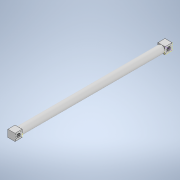
# Autodesk Inventor part: wał
Saved by Autodesk Inventor 2022 (Build 260153000, 153)
## iProperties
Created: 2023-04-25
Part Number: wał
Material: Ogólny
Document SubType Name: Modeling
Designer: nosal
Density: 1 g/cm^3
Appearance: Domyślna
Author: nosal
Autodesk Inventor part; units mm, degrees
ref_plane "YZ Plane" through (0, 0, 0) normal (1, 0, 0) x (0, 1, 0)
ref_plane "XZ Plane" through (0, 0, 0) normal (0, 1, 0) x (-1, 0, 0)
ref_plane "XY Plane" through (0, 0, 0) normal (0, 0, 1) x (1, 0, 0)
sketch "Szkic1" plane through (0, 0, 0) normal (0, 0, 1) x (1, 0, 0)
  circle A0 centre (0, 0) radius 4
  dimension "d0" = 8
  constraints: 1 centre point, 1 coincident
  measures "d0" diameter of A0
extrude "Wyciągnięcie proste1" add sketch "Szkic1" along normal blind 160
sketch "Szkic2" plane through (0, 0, 160) normal (0, 0, 1) x (1, 0, 0)
  line L0 (4, -4) -> (-4, -4)
  line L1 (-4, -4) -> (-4, 4)
  line L2 (-4, 4) -> (4, 4)
  line L3 (4, 4) -> (4, -4)
  line L4 (4, -4) -> (-4, 4) construction
  line L5 (-4, -4) -> (4, 4) construction
  point P0 (0, 0)
  dimension "d3" = 8
  dimension "d4" = 8
  constraints: 12 end point, 2 midpoint, 2 parallel, 1 horizontal, 1 perpendicular
  measures "d3" distance of L1.end L2.end
  measures "d4" distance of L0.end L1.end
extrude "Wyciągnięcie proste2" add sketch "Szkic2" along normal blind 8
sketch "Szkic3" plane through (0, 0, 0) normal (0, 0, -1) x (-1, 0, 0)
  line L0 (4, -4) -> (-4, -4) projected
  line L1 (4, 4) -> (-4, 4)
  line L2 (-4, 4) -> (-4, -4)
  line L3 (-4, -4) -> (4, -4)
  line L4 (4, -4) -> (4, 4)
  line L5 (4, 4) -> (-4, -4) construction
  line L6 (-4, 4) -> (4, -4) construction
  point P0 (0, 0)
  constraints: 12 end point, 2 midpoint, 2 parallel, 1 horizontal, 1 perpendicular
extrude "Wyciągnięcie proste3" add sketch "Szkic3" along normal blind 8
sketch "Szkic4" plane through (4, 0, 0) normal (1, 0, 0) x (0, 0, -1)
  line L0 (0, -4) -> (8, -4) construction
  line L1 (8, -4) -> (0, 3.9612) construction
  line L2 (0, 0) -> (0, -4) construction
  line L3 (8, -4) -> (8, 4) construction
  line L4 (0, -4) -> (8, 4) construction
  line L5 (-160, 0) -> (-160, -4) construction
  line L6 (-168, 4) -> (-168, -4) construction
  line L7 (-160, -4) -> (-168, 4) construction
  line L8 (-168, 4) -> (-168, -4) construction
  line L9 (-168, -4) -> (-160, 4) construction
  constraints: 10 end point, 1 collinear, 1 perpendicular
sketch "Szkic5" plane through (4, 0, 0) normal (1, 0, 0) x (0, 0, -1)
  point P0 (0, 0)
  point P1 (3.9975, -0.0288)
hole "Otwór1" at (4, -0.0288, -3.9975) direction (-1, 0, 0) diameter 4.134 end through all thread size "M5x0.8" class "6H" standard "ANSI Metric M Profile"
sketch "Szkic6" plane through (4, -4, 160) normal (1, 0, 0) x (0, 0, -1)
  point P0 (160, 4)
  point P1 (-4, 3.9995)
hole "Otwór2" at (4, -0.0005, 164) direction (-1, 0, 0) diameter 4.134 end through all thread size "M5x0.8" class "6H" standard "ANSI Metric M Profile"
